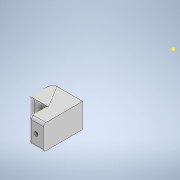
# Autodesk Inventor part: 3D_print_actuator
Saved by Autodesk Inventor 2021 (Build 250183000, 183)
## iProperties
Created: 2021-04-12
Part Number: 3D_print_actuator
Material: Generic
Document SubType Name: Modeling
Designer: Charlie
Density: 1 g/cm^3
Appearance: Default
Author: Charlie
Autodesk Inventor part; units mm, degrees
ref_plane "YZ Plane" through (0, 0, 0) normal (1, 0, 0) x (0, 1, 0)
ref_plane "XY Plane" through (0, 0, 0) normal (0, 0, 1) x (1, 0, 0)
sketch "Sketch1" plane through (0, 0, 0) normal (0, 1, 0) x (-1, 0, 0)
  line L0 (0, -106) -> (0, 94)
  line L1 (0, -106) -> (21, -106) construction
  line L2 (30, -97) -> (30, -97) construction
  line L3 (0, -106) -> (12, -106) construction
  line L4 (21, -88) -> (12, -88) construction
  line L5 (12, -88) -> (12, -86)
  line L6 (12, -106) -> (21, -106)
  line L7 (30, -88) -> (21, -88) construction
  line L8 (30, -88) -> (30, -106) construction
  arc A0 (21, -106) -> (30, -97) centre (21, -97) ccw
  arc A1 (30, -97) -> (21, -88) centre (21, -97) ccw
  line L9 (21, -106) -> (30, -106) construction
  line L10 (21, -88) -> (12, -88)
  line L11 (12, -68) -> (12, -66)
  arc A2 (21, -86) -> (30, -77) centre (21, -77) ccw
  arc A3 (30, -77) -> (21, -68) centre (21, -77) ccw
  line L12 (0, -86) -> (21, -86) construction
  line L13 (21, -68) -> (12, -68) construction
  line L14 (21, -68) -> (12, -68)
  line L15 (12, -86) -> (21, -86)
  line L16 (12, -48) -> (12, -46)
  arc A4 (21, -66) -> (30, -57) centre (21, -57) ccw
  arc A5 (30, -57) -> (21, -48) centre (21, -57) ccw
  line L17 (0, -66) -> (21, -66) construction
  line L18 (21, -48) -> (12, -48) construction
  line L19 (21, -48) -> (12, -48)
  line L20 (12, -66) -> (21, -66)
  line L21 (12, -28) -> (12, -26)
  arc A6 (21, -46) -> (30, -37) centre (21, -37) ccw
  arc A7 (30, -37) -> (21, -28) centre (21, -37) ccw
  line L22 (0, -46) -> (21, -46) construction
  line L23 (21, -28) -> (12, -28) construction
  line L24 (21, -28) -> (12, -28)
  line L25 (12, -46) -> (21, -46)
  line L26 (12, -8) -> (12, -6)
  arc A8 (21, -26) -> (30, -17) centre (21, -17) ccw
  arc A9 (30, -17) -> (21, -8) centre (21, -17) ccw
  line L27 (0, -26) -> (21, -26) construction
  line L28 (21, -8) -> (12, -8) construction
  line L29 (21, -8) -> (12, -8)
  line L30 (12, -26) -> (21, -26)
  line L31 (12, 12) -> (12, 14)
  arc A10 (21, -6) -> (30, 3) centre (21, 3) ccw
  arc A11 (30, 3) -> (21, 12) centre (21, 3) ccw
  line L32 (0, -6) -> (21, -6) construction
  line L33 (21, 12) -> (12, 12) construction
  line L34 (21, 12) -> (12, 12)
  line L35 (12, -6) -> (21, -6)
  line L36 (12, 32) -> (12, 34)
  arc A12 (21, 14) -> (30, 23) centre (21, 23) ccw
  arc A13 (30, 23) -> (21, 32) centre (21, 23) ccw
  line L37 (0, 14) -> (21, 14) construction
  line L38 (21, 32) -> (12, 32) construction
  line L39 (21, 32) -> (12, 32)
  line L40 (12, 14) -> (21, 14)
  line L41 (12, 52) -> (12, 54)
  arc A14 (21, 34) -> (30, 43) centre (21, 43) ccw
  arc A15 (30, 43) -> (21, 52) centre (21, 43) ccw
  line L42 (0, 34) -> (21, 34) construction
  line L43 (21, 52) -> (12, 52) construction
  line L44 (21, 52) -> (12, 52)
  line L45 (12, 34) -> (21, 34)
  line L46 (12, 72) -> (12, 74)
  arc A16 (21, 54) -> (30, 63) centre (21, 63) ccw
  arc A17 (30, 63) -> (21, 72) centre (21, 63) ccw
  line L47 (0, 54) -> (21, 54) construction
  line L48 (21, 72) -> (12, 72) construction
  line L49 (21, 72) -> (12, 72)
  line L50 (12, 54) -> (21, 54)
  line L51 (12, 92) -> (12, 94)
  arc A18 (21, 74) -> (30, 83) centre (21, 83) ccw
  arc A19 (30, 83) -> (21, 92) centre (21, 83) ccw
  line L52 (0, 74) -> (21, 74) construction
  line L53 (21, 92) -> (12, 92) construction
  line L54 (21, 92) -> (12, 92)
  line L55 (12, 74) -> (21, 74)
  line L56 (0, 94) -> (0, 106)
  line L57 (0, 106) -> (6, 106)
  line L58 (12, 100) -> (12, 94)
  line L59 (12, -106) -> (0, -106)
  line L60 (12, 100) -> (12, 106)
  line L61 (12, 106) -> (6, 106)
  line L62 (0, -106) -> (64, -106)
  line L63 (64, -106) -> (64, 74)
  line L64 (64, 74) -> (0, 74)
  line L65 (0, 74) -> (0, -106)
  point P0 (0, 0)
  point P1 (30, -86)
  point P2 (30, -68)
  point P3 (30, -66)
  point P4 (30, -48)
  point P5 (30, -46)
  point P6 (30, -28)
  point P7 (30, -26)
  point P8 (30, -8)
  point P9 (30, -6)
  point P10 (30, 12)
  point P11 (30, 14)
  point P12 (30, 32)
  point P13 (30, 34)
  point P14 (30, 52)
  point P15 (30, 54)
  point P16 (30, 72)
  point P17 (30, 74)
  point P18 (30, 92)
  point P19 (30, -97)
  point P20 (21, 74)
  point P21 (0, 74)
  dimension "d0" = 94
  dimension "d1" = 110.1635
  dimension "d2" = 18
  dimension "d3" = 106.6771
  dimension "d4" = 2
  dimension "d5" = 9
  dimension "d6" = 9
  dimension "d11" = 20
  dimension "d16" = 12
  dimension "d17" = 12
  dimension "d60" = 64
  constraints: 132 end point, 40 point on circle, 34 point on line, 20 centre point, 6 perpendicular, 5 equal length, 5 vertical, 4 horizontal, 4 tangent, 1 collinear, 169 other
  measures "d0" distance of point (0, 0) L0.end
  measures "d1" distance of point (0, 0) L8.end
  measures "d2" distance of L8.end L7.start
  measures "d3" distance of point (0, 0) L3.end
  measures "d4" distance of L4.end L5.end
  measures "d5" radius of A0
  measures "d6" radius of A1
  measures "d11" distance of L4.end L11.start
  measures "d16" distance of L0.end L56.end
  measures "d17" distance of L56.end L60.end
  measures "d60" distance of L64.end L63.end
extrude "Extrusion1" add sketch "Sketch1" along normal blind 20 contours L0 L64 L46 L49 A17 A16 L50 L41 L44 A15 A14 L45 L36 L39 A13 A12 L40 L31 L34 A11 A10 L35 L26 L29 A9 A8 L30 L21 L24 A7 A6 L25 L16 L19 A5 A4 L20 L11 L14 A3 A2 L15 L5 L10 A1 A0 L6 L59 | L0 L56 L57 L61 L60 L58 L51 L54 A19 A18 L55 L64
sketch "Sketch2" plane through (0, 0, -106) normal (0, 0, -1) x (-1, 0, 0)
  line L0 (30, 20) -> (21, 20) construction
  line L1 (21, 20) -> (0, 20)
  line L2 (0, 20) -> (0, 0)
  line L3 (0, 0) -> (21, 0)
  line L4 (30, 9) -> (30, 11)
  line L5 (30, 20) -> (0, 0) construction
  arc A0 (30, 11) -> (21, 20) centre (21, 11) ccw
  arc A1 (21, 0) -> (30, 9) centre (21, 9) ccw
  line L6 (5.5, -4) -> (24.5, -4)
  line L7 (24.5, -4) -> (24.5, 24)
  line L8 (24.5, 24) -> (5.5, 24)
  line L9 (5.5, 24) -> (5.5, -4)
  line L10 (5.5, -4) -> (24.5, 24) construction
  line L11 (24.5, -4) -> (5.5, 24) construction
  line L12 (24.5, 24) -> (37.5, 24)
  line L13 (37.5, 24) -> (37.5, 0)
  line L14 (37.5, 0) -> (24.5, -4)
  point P0 (0, 0)
  point P1 (30, 0)
  point P2 (15, 10)
  point P3 (5.5, 0)
  point P4 (5.5, 20)
  dimension "d21" = 30
  dimension "d22" = 20
  dimension "d23" = 9
  dimension "d24" = 9
  dimension "d25" = 19
  dimension "d26" = 28
  dimension "d65" = 13
  constraints: 28 end point, 4 parallel, 4 point on circle, 4 point on line, 4 tangent, 3 horizontal, 3 midpoint, 3 perpendicular, 2 centre point
  measures "d21" distance of point (0, 0) point (30, 0)
  measures "d22" distance of L1.end point (0, 0)
  measures "d23" radius of A0
  measures "d24" radius of A1
  measures "d25" distance of L8.end L7.end
  measures "d26" distance of L7.end L6.end
  measures "d65" distance of L7.end L12.end
extrude "Extrusion2" cut sketch "Sketch2" against normal blind 200 contours L1 L9 L8 L7 A0 | L7 L12 L13 L14 A1 L4 A0 | L3 A1 L7 L6 L9
shell "Shell2" thickness 1 removed faces 1 at (-8, 6.6667, 106)
sketch "Sketch7" plane through (-12, 0, 106) normal (0, 0, 1) x (1, 0, 0)
  line L0 (0, 20) -> (12, 20) projected
  line L1 (0, 0) -> (12, 0)
  line L2 (12, 0) -> (12, 20)
  line L3 (12, 20) -> (0, 20)
  line L4 (0, 20) -> (0, 0)
  circle A0 centre (6, 10) radius 1.5
  point P0 (12, 0)
  dimension "d46" = 3
  dimension "d66" = 6
  dimension "d67" = 10
  constraints: 8 end point, 2 parallel, 1 centre point, 1 horizontal, 1 perpendicular
  measures "d46" diameter of A0
  measures "d66" distance from line of L4 A0.centre
  measures "d67" distance from line of L0 A0.centre
extrude "Extrusion5" add sketch "Sketch7" against normal blind 8 contours L0 L2 L1 L4 | A0
fillet "Fillet2" radius 2 5 edges at (-12, 20, 99) (-12, 10, 106) (-12, 0, 99) (-6, 0, 106) (-6, 20, 106)
extrude "Extrusion6" cut sketch "Sketch7" against normal blind 2 contours A0
sketch "Sketch8" plane through (0, 0, 0) normal (1, 0, 0) x (0, 1, 0)
  line L0 (0, -88) -> (20, -88) projected
  line L1 (0, -86) -> (20, -86) projected
  line L2 (0, 9) -> (20, 9)
  line L3 (20, 9) -> (20, 10)
  line L4 (20, 10) -> (0, 10)
  line L5 (0, 10) -> (0, 9)
  line L6 (0, 19) -> (20, 19)
  line L7 (20, 20) -> (0, 20)
  line L8 (20, 19) -> (20, 20)
  line L9 (0, 20) -> (0, 19)
  line L10 (0, 29) -> (20, 29)
  line L11 (20, 30) -> (0, 30)
  line L12 (20, 29) -> (20, 30)
  line L13 (0, 30) -> (0, 29)
  line L14 (0, 39) -> (20, 39)
  line L15 (20, 40) -> (0, 40)
  line L16 (20, 39) -> (20, 40)
  line L17 (0, 40) -> (0, 39)
  line L18 (0, 49) -> (20, 49)
  line L19 (20, 50) -> (0, 50)
  line L20 (20, 49) -> (20, 50)
  line L21 (0, 50) -> (0, 49)
  line L22 (0, 59) -> (20, 59)
  line L23 (20, 60) -> (0, 60)
  line L24 (20, 59) -> (20, 60)
  line L25 (0, 60) -> (0, 59)
  line L26 (0, 69) -> (20, 69)
  line L27 (20, 70) -> (0, 70)
  line L28 (20, 69) -> (20, 70)
  line L29 (0, 70) -> (0, 69)
  line L30 (0, 79) -> (20, 79)
  line L31 (20, 80) -> (0, 80)
  line L32 (20, 79) -> (20, 80)
  line L33 (0, 80) -> (0, 79)
  line L34 (0, 89) -> (20, 89)
  line L35 (20, 90) -> (0, 90)
  line L36 (20, 89) -> (20, 90)
  line L37 (0, 90) -> (0, 89)
  point P0 (0, 0)
  dimension "d51" = 10
  constraints: 72 end point, 2 parallel, 1 collinear, 1 horizontal, 1 perpendicular, 1 vertical, 65 other
  measures "d51" distance of L2.start L6.start
extrude "Extrusion7" [suppressed]
ref_plane "Work Plane1" through (-21, 0, 91.5) normal (0, 0, 1) x (1, 0, 0)
sketch "Sketch4" plane through (-21, 0, 91.5) normal (0, 0, 1) x (1, 0, 0)
  line L0 (0, 0) -> (0, 20) projected
  line L1 (0, 0) -> (12, 20) construction
  circle A0 centre (6, 10) radius 2 construction
  line L2 (5, 6.5) -> (1, 6.5)
  line L3 (1, 6.5) -> (1, 13.5)
  line L4 (1, 13.5) -> (5, 13.5)
  line L5 (5, 13.5) -> (5, 6.5)
  line L6 (5, 6.5) -> (1, 13.5) construction
  line L7 (1, 6.5) -> (5, 13.5) construction
  point P0 (21, 0)
  point P1 (3, 10)
  point P2 (1, 10)
  point P3 (5, 8.2679)
  dimension "d31" = 4
  dimension "d58" = 4
  dimension "d59" = 7
  constraints: 14 end point, 3 midpoint, 2 parallel, 1 centre point, 1 horizontal, 1 perpendicular
  measures "d31" diameter of A0
  measures "d58" distance of L3.end L4.end
  measures "d59" distance of L2.end L3.end
extrude "Extrusion3" [suppressed]
extrude "Extrusion8" cut sketch "Sketch1" along normal blind 20 contours L0 L64 L46 L49 A17 A16 L50 L41 L44 A15 A14 L45 L36 L39 A13 A12 L40 L31 L34 A11 A10 L35 L26 L29 A9 A8 L30 L21 L24 A7 A6 L25 L16 L19 A5 A4 L20 L11 L14 A3 A2 L15 L5 L10 A1 A0 L6 L59 | L55 L64 L63 L62 A0 A1 L10 L5 L15 A2 A3 L14 L11 L20 A4 A5 L19 L16 L25 A6 A7 L24 L21 L30 A8 A9 L29 L26 L35 A10 A11 L34 L31 L40 A12 A13 L39 L36 L45 A14 A15 L44 L41 L50 A16 A17 L49 L46
sketch "Sketch9" plane through (0, 0, 74) normal (0, 0, -1) x (-1, 0, 0)
  line L0 (11, 19) -> (1, 19) projected
  line L1 (11, 19) -> (0, 19)
  line L2 (0, 19) -> (0, 0)
  line L3 (0, 0) -> (11, 0)
  line L4 (11, 0) -> (11, 19)
  constraints: 8 end point, 2 parallel, 1 horizontal, 1 perpendicular
extrude "Extrusion9" add sketch "Sketch9" against normal blind 1
ref_plane "Work Plane2" through (0, 10, 0) normal (0, 1, 0) x (-1, 0, 0)
sketch "Sketch10" plane through (0, 20, 0) normal (0, 1, 0) x (1, 0, 0)
  line L0 (-10, -104) -> (-10, -92) construction
  line L1 (-21, -92) -> (-21, -74) construction
  line L2 (-10, -92) -> (-21, -74) construction
  point P0 (0, 0)
  constraints: 2 end point
sketch "Sketch6" plane through (0, 10, 0) normal (0, 1, 0) x (-1, 0, 0)
  line L0 (40.7593, 109.726) -> (-19.2407, 109.726)
  line L1 (-19.2407, 109.726) -> (-19.2407, -3.5286)
  line L2 (-19.2407, -3.5286) -> (40.7593, -3.5286)
  line L3 (40.7593, -3.5286) -> (40.7593, 109.726)
  point P0 (0, 0)
  dimension "d36" = 113.2546
  dimension "d37" = 60
  constraints: 8 end point, 2 parallel, 1 horizontal, 1 perpendicular
  measures "d36" distance of L2.end L0.start
  measures "d37" distance of L1.end L2.end
body "Solid1"
